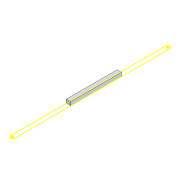
# Autodesk Inventor part: Part_13_p3
Saved by Autodesk Inventor 2022 (Build 260153000, 153)
## iProperties
Created: 2022-04-26
Part Number: Part_13_p3
Material: Generic
Document SubType Name: Modeling
Designer: dell
Density: 1 g/cm^3
Appearance: Default
Author: dell
Autodesk Inventor part; units mm, degrees
ref_plane "YZ Plane" through (0, 0, 0) normal (1, 0, 0) x (0, 1, 0)
ref_plane "XZ Plane" through (0, 0, 0) normal (0, 1, 0) x (-1, 0, 0)
ref_plane "XY Plane" through (0, 0, 0) normal (0, 0, 1) x (1, 0, 0)
sketch "Sketch1" plane through (0, 0, 0) normal (0, 1, 0) x (-1, 0, 0)
  line L0 (0, 0) -> (0, -351.981) construction
  line L1 (-5, 0) -> (-5, -351.981)
  line L2 (5, -351.981) -> (5, 0)
  arc A0 (5, 0) -> (-5, 0) centre (0, 0) ccw
  arc A1 (-5, -351.981) -> (5, -351.981) centre (0, -351.981) ccw
  circle A2 centre (0, 0) radius 1.5
  circle A3 centre (0, -351.981) radius 1.5
  point P0 (0, -175.9905)
  dimension "d0" = 351.981
  dimension "d1" = 10
  dimension "d2" = 3
  dimension "d3" = 3
  constraints: 8 end point, 4 centre point, 4 point on circle, 4 tangent, 2 coincident, 1 midpoint, 1 parallel, 1 vertical
  measures "d0" distance of L0.start L0.end
  measures "d1" diameter of A1
  measures "d2" diameter of A2
  measures "d3" diameter of A3
extrude "Extrusion1" add sketch "Sketch1" along normal blind 8
sketch "Sketch2" plane through (0, 0, 0) normal (0, -1, 0) x (1, 0, 0)
  arc A0 (-5, -351.981) -> (5, -351.981) centre (0, -351.981) ccw projected
  line L0 (5, 0) -> (5, -351.981) projected
  arc A1 (5, 0) -> (-5, 0) centre (0, 0) ccw projected
  line L1 (-5, -351.981) -> (-5, 0) projected
  circle A2 centre (0, -351.981) radius 1.5 projected
  circle A3 centre (0, 0) radius 1.5 projected
sketch "Sketch3" plane through (0, 8, 0) normal (0, 1, 0) x (1, 0, 0)
  line L0 (-27.6747, 127.2679) -> (44.1637, 127.2679)
  line L1 (44.1637, 127.2679) -> (44.1637, -33.2034)
  line L2 (44.1637, -33.2034) -> (-27.6747, -33.2034)
  line L3 (-27.6747, -33.2034) -> (-27.6747, 127.2679)
  line L4 (-64.8326, 381.1064) -> (113.525, 381.1064)
  line L5 (113.525, 381.1064) -> (113.525, -69.742)
  line L6 (113.525, -69.742) -> (-64.8326, -69.742)
  line L7 (-64.8326, -69.742) -> (-64.8326, 381.1064)
  line L8 (-27.6747, 127.2679) -> (44.1637, 127.2679)
  line L9 (44.1637, 127.2679) -> (44.1637, 242.6063)
  line L10 (44.1637, 242.6063) -> (-27.6747, 242.6063)
  line L11 (-27.6747, 242.6063) -> (-27.6747, 127.2679)
  point P0 (0, 0)
  constraints: 24 end point, 6 parallel, 3 horizontal, 3 perpendicular
extrude "Extrusion2" cut sketch "Sketch3" against normal blind 10 contours L0 L1 L2 L3 | L4 L5 L6 L7
body "Solid1"
